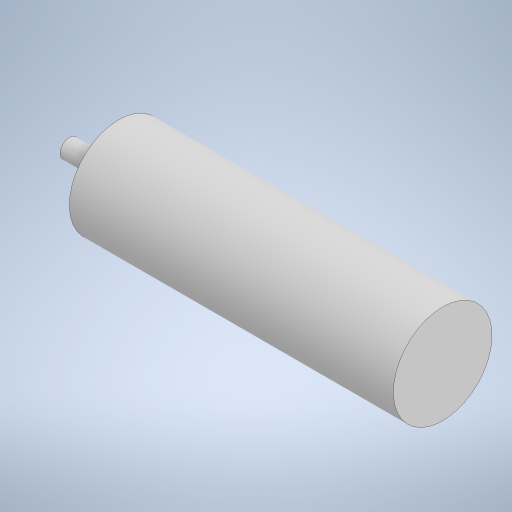
# Autodesk Inventor part: planetary motor
Saved by Autodesk Inventor 2023 (Build 270158000, 158)
## iProperties
Created: 2023-01-11
Part Number: planetary motor
Material: Generic
Document SubType Name: Modeling
Designer: victo
Density: 1 g/cm^3
Appearance: Default
Author: victo
Autodesk Inventor part; units mm, degrees
ref_plane "YZ Plane" through (0, 0, 0) normal (1, 0, 0) x (0, 1, 0)
ref_plane "XZ Plane" through (0, 0, 0) normal (0, 1, 0) x (-1, 0, 0)
ref_plane "XY Plane" through (0, 0, 0) normal (0, 0, 1) x (1, 0, 0)
sketch "Sketch2" plane through (0, 0, 0) normal (0, 0, 1) x (1, 0, 0)
  line L0 (-19.3282, 17.8384) -> (85.6718, 17.8384)
  line L1 (85.6718, 17.8384) -> (85.6718, 1.8384)
  line L2 (-19.3282, 4.8384) -> (-35.3282, 4.8384)
  line L3 (-35.3282, 4.8384) -> (-35.3282, 1.8384)
  line L4 (-35.3282, 1.8384) -> (-19.3282, 1.8384)
  line L5 (-19.3282, 1.8384) -> (-19.3282, 4.8384)
  line L6 (-54.2545, 1.8384) -> (116.821, 1.8384)
  line L7 (-19.3282, 1.8384) -> (-19.3282, 4.8384)
  line L8 (-19.3282, 1.8384) -> (-19.3282, 17.8384)
  point P0 (0, 0)
  dimension "d1" = 16
  dimension "d3" = 3
  dimension "d4" = 16
  dimension "d5" = 105
  constraints: 18 end point, 4 parallel, 3 horizontal, 2 perpendicular, 2 point on line, 1 collinear
  measures "d1" distance of L0.end L1.end
  measures "d3" distance of L3.end L2.end
  measures "d4" distance of L2.start L2.end
  measures "d5" distance of L0.start L0.end
revolve "Revolution1" add sketch "Sketch2" angle 360 about axis through (-54.2545, 1.8384, 0) along (1, 0, 0)
body "Solid1"
